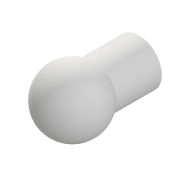
# Autodesk Inventor part: endEffector
Saved by Autodesk Inventor 2021 (Build 250183000, 183)
## iProperties
Created: 2020-08-17
Part Number: endEffector
Material: Generic
Document SubType Name: Modeling
Designer: Derm
Density: 1 g/cm^3
Appearance: Default
Author: Derm
Autodesk Inventor part; units mm, degrees
ref_plane "YZ Plane" through (0, 0, 0) normal (1, 0, 0) x (0, 1, 0)
ref_plane "XZ Plane" through (0, 0, 0) normal (0, 1, 0) x (-1, 0, 0)
ref_plane "XY Plane" through (0, 0, 0) normal (0, 0, 1) x (1, 0, 0)
sketch "Sketch1" plane through (0, 0, 0) normal (0, 0, 1) x (1, 0, 0)
  circle A0 centre (0, 0) radius 25.56 projected
  point P0 (0, 0)
extrude "Extrusion1" add sketch "Sketch1" along normal blind 50.8
sketch "Sketch2" plane through (0, 0, 0) normal (1, 0, 0) x (0, 1, 0)
  line L0 (25.56, 0) -> (25.56, 50.8) projected
  line L1 (0, 0) -> (0, 109.3667)
  arc A0 (25.56, 50.8) -> (0, 109.3667) centre (0, 74.5058) ccw
  line L2 (25.56, 50.8) -> (0, 50.8)
  line L3 (25.56, 50.8) -> (-25.56, 50.8) projected
  point P0 (0, 50.8)
  constraints: 4 end point, 2 point on circle, 1 centre point, 1 midpoint, 1 point on line, 1 vertical
revolve "Revolution1" add sketch "Sketch2" angle 360 about axis through (0, 0, 0) along (0, 0, 1)
body "Solid1"
